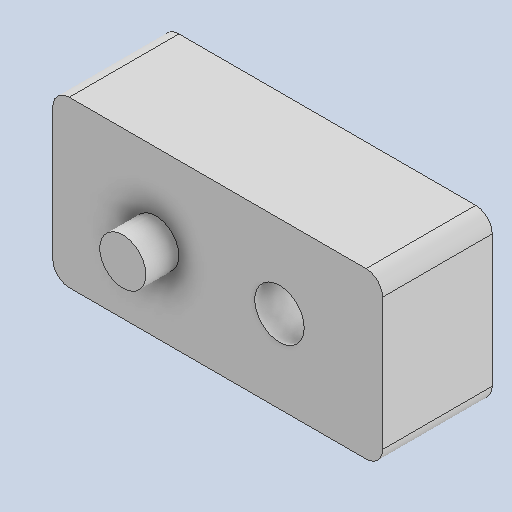
# Autodesk Inventor part: PWR_PCBA_HeatSink
Saved by Autodesk Inventor 2022 (Build 260153000, 153)
## iProperties
Created: 2021-01-19
Part Number: PWR_PCBA_HeatSink
Material: Generic
Document SubType Name: Modeling
Designer: lgnds
Density: 1 g/cm^3
Appearance: Default
Author: lgnds
Autodesk Inventor part; units mm, degrees
ref_plane "YZ Plane" through (0, 0, 0) normal (1, 0, 0) x (0, 1, 0)
ref_plane "XZ Plane" through (0, 0, 0) normal (0, 1, 0) x (-1, 0, 0)
ref_plane "XY Plane" through (0, 0, 0) normal (0, 0, 1) x (1, 0, 0)
sketch "Sketch1" plane through (0, 0, 0) normal (0, 0, 1) x (1, 0, 0)
  line L0 (-10, -5) -> (10, -5)
  line L1 (10, -5) -> (10, 5)
  line L2 (10, 5) -> (-10, 5)
  line L3 (-10, 5) -> (-10, -5)
  line L4 (-10, -5) -> (10, 5) construction
  line L5 (10, -5) -> (-10, 5) construction
  line L6 (-14, 0) -> (14, 0) construction
  circle A0 centre (3.75, 0) radius 1.5
  point P0 (0, 0)
  dimension "d0" = 20
  dimension "d1" = 10
  dimension "d2" = 3
  dimension "d3" = 3.75
  constraints: 12 end point, 2 midpoint, 2 parallel, 1 centre point, 1 horizontal, 1 perpendicular, 1 point on line
  measures "d0" distance between parallel lines of L1 L3
  measures "d1" distance of L0.end L1.end
  measures "d2" diameter of A0
  measures "d3" distance of point (0, 0) A0.centre
extrude "Extrusion1" add sketch "Sketch1" along normal blind 6.65
sketch "Sketch2" plane through (0, 0, 6.65) normal (0, 0, 1) x (1, 0, 0)
  line L0 (-14, 0) -> (14, 0) projected
  circle A0 centre (-3.75, 0) radius 1.4
  point P0 (0, 0)
  dimension "d6" = 2.8
  dimension "d7" = 3.75
  constraints: 1 centre point, 1 point on line
  measures "d6" diameter of A0
  measures "d7" distance of point (0, 0) A0.centre
extrude "Extrusion2" add sketch "Sketch2" along normal blind 2
fillet "Fillet2" radius 1 4 edges at (10, -5, 3.325) (10, 5, 3.325) (-10, -5, 3.325) (-10, 5, 3.325)
body "Solid1"
